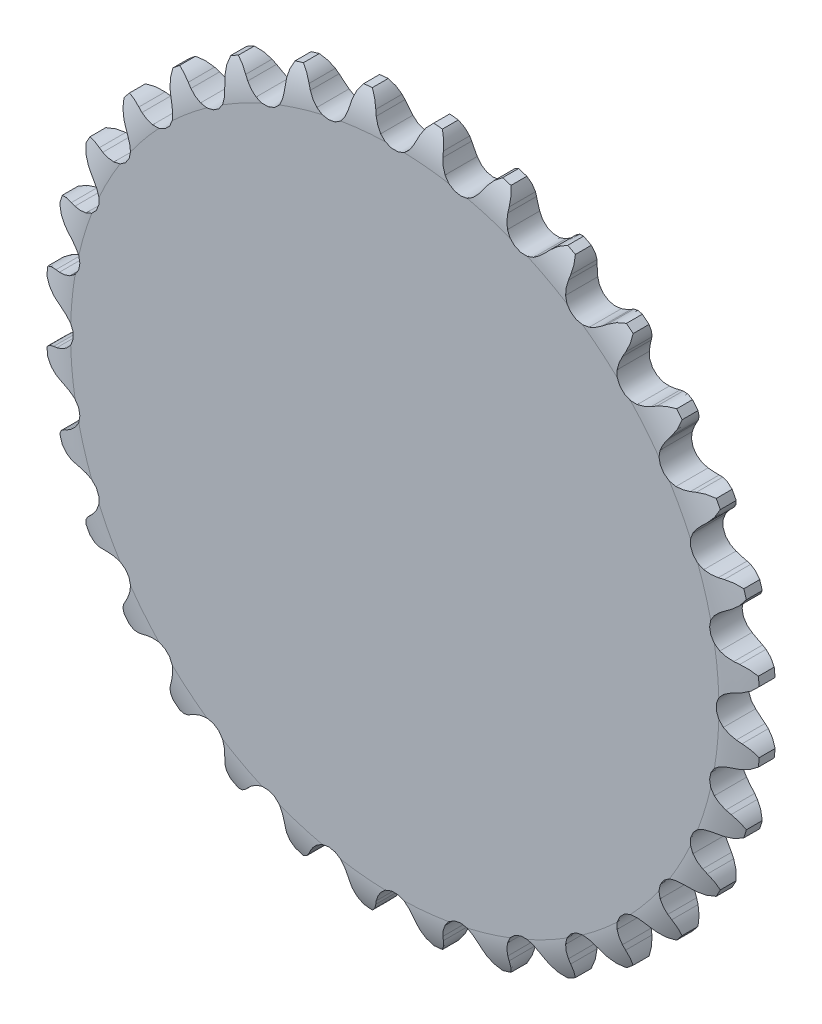
# Autodesk Inventor part: Roller Chain Sprocket1
Saved by Autodesk Inventor 2016 SP1 (Build 200210100, 210)
## iProperties
Created: 2016-02-12
Part Number: Roller Chain Sprocket1
Material: Steel
Document SubType Name: Modeling
Designer: steele
Density: 1 g/cm^3
Appearance: Steel
CustomPartVersion: 1
Author: steele
Autodesk Inventor part; units mm, degrees
ref_plane "YZ Plane" through (0, 0, 0) normal (1, 0, 0) x (0, 1, 0)
ref_plane "XZ Plane" through (0, 0, 0) normal (0, 1, 0) x (-1, 0, 0)
ref_plane "XY Plane" through (0, 0, 0) normal (0, 0, 1) x (1, 0, 0)
sketch "Theoretical Tooth Profile" plane through (0, 0, 0) normal (0, 0, 1) x (1, 0, 0)
  circle A0 centre (0, 0) radius 32.3923 construction
  line L0 (0, 0) -> (0, 32.3923) construction
  line L1 (0, 0) -> (6.3194, 31.7699) construction
  circle A1 centre (0, 0) radius 34.1413
  arc A2 (-1.3578, 31.3738) -> (1.3578, 31.3738) centre (0, 32.3923) ccw
  line L2 (0, 32.3923) -> (6.3194, 31.7699) construction
  line L3 (0, 32.3923) -> (2.1131, 33.9774) construction
  line L4 (2.1131, 33.9774) -> (-1.9477, 32.449) construction
  arc A3 (2.9335, 34.0151) -> (2.1088, 32.877) centre (4.6005, 31.9392) ccw
  arc A4 (-2.1088, 32.877) -> (-2.9335, 34.0151) centre (-4.6005, 31.9392) ccw
  line L5 (-4.6005, 31.9392) -> (-2.1088, 32.877) construction
  arc A5 (-1.9477, 32.449) -> (-1.3578, 31.3738) centre (2.1131, 33.9774) ccw
  line L6 (-1.9477, 32.449) -> (-2.1088, 32.877)
  arc A6 (1.3578, 31.3738) -> (1.9477, 32.449) centre (-2.1131, 33.9774) ccw
  line L7 (2.1088, 32.877) -> (1.9477, 32.449)
  line L8 (0, 0) -> (3.3464, 33.9769) construction
  point P0 (3.1597, 32.0811)
  dimension "d0" = 64.7846
  dimension "d2" = 11.25
  dimension "d3" = 1.6973
  dimension "d10" = 126.875
  dimension "d11" = 16.25
  dimension "d12" = 2.6416
  dimension "d13" = 4.339
  dimension "d14" = 4.6228
  dimension "d23" = 1.905
  constraints: 18 end point, 15 point on circle, 7 centre point, 3 coincident, 3 point on line, 3 symmetric about line, 3 tangent, 1 equal radius, 1 midpoint, 1 parallel, 1 vertical, 1 other
  measures "d0" diameter of A0
  measures "d2" angle of L1 L0
  measures "d3" radius of A2
  measures "d10" angle of L3 L0
  measures "d11" angle of L4 L3
  measures "d12" distance of L2.start L3.end
  measures "d13" distance of L3.end L4.end
  measures "d14" distance of A3.centre L0.end
  measures "d23" distance from line of L8.end L2
sketch "Tooth Profile" plane through (0, 0, 0) normal (0, 0, 1) x (1, 0, 0)
  circle A0 centre (0, 0) radius 34.1413 projected
  line L0 (0, 0) -> (0, 32.3923) construction
  line L1 (0, 32.3923) -> (1.5803, 31.7728) construction
  arc A1 (-1.5803, 31.7728) -> (1.5803, 31.7728) centre (0, 32.3923) ccw
  line L2 (-1.5803, 31.7728) -> (0, 32.3923) construction
  arc A2 (-1.5803, 31.7728) -> (-2.7217, 34.0327) centre (-14.1231, 26.8557) ccw
  arc A3 (2.7217, 34.0327) -> (1.5803, 31.7728) centre (14.1231, 26.8557) ccw
  dimension "d44" = 137.188
  dimension "d45" = 1.6973
  dimension "d46" = 13.4722
  constraints: 8 point on circle, 7 end point, 3 centre point, 2 tangent, 1 coincident, 1 equal radius, 1 symmetric about line, 1 vertical
  measures "d44" angle of L1 L2
  measures "d45" radius of A1
  measures "d46" radius of A3
sketch "Section Profile" plane through (0, 0, 0) normal (1, 0, 0) x (0, 1, 0)
  line L0 (34.1413, 0) -> (-34.1413, 0) projected
  line L1 (28.4263, 1.5526) -> (-28.4263, 1.5526)
  line L2 (-28.4263, 1.5526) -> (-28.4263, -1.5526)
  line L3 (-28.4263, -1.5526) -> (28.4263, -1.5526)
  line L4 (28.4263, -1.5526) -> (28.4263, 1.5526)
  line L5 (28.4263, 1.5526) -> (34.1413, 1.5526) construction
  line L6 (34.1413, 1.5526) -> (34.1413, -1.5526) construction
  line L7 (34.1413, -1.5526) -> (28.4263, -1.5526) construction
  line L8 (28.4263, -1.5526) -> (28.4263, 1.5526)
  arc A0 (34.1413, 0.7588) -> (30.9655, 1.5526) centre (30.9655, -5.1975) ccw
  arc A1 (30.9655, -1.5526) -> (34.1413, -0.7588) centre (30.9655, 5.1975) ccw
  line L9 (30.9655, 1.5526) -> (0, 1.5526)
  line L10 (0, 1.5526) -> (0, -1.5526)
  line L11 (0, -1.5526) -> (30.9655, -1.5526)
  line L12 (0, 1.5526) -> (0, -1.5526)
  line L13 (34.1413, 0.7588) -> (34.1413, -0.7588)
  point P0 (0, 0)
  point P1 (0, 0)
  dimension "d30" = 3.1052
  dimension "d31" = 56.8526
  dimension "d32" = 3.1052
  dimension "d33" = 0.7937
  dimension "d34" = 6.75
  dimension "d43" = 1.5526
  constraints: 26 end point, 7 midpoint, 5 perpendicular, 4 parallel, 4 point on circle, 3 point on line, 3 symmetric about line, 2 centre point, 2 horizontal, 2 tangent, 1 collinear, 1 other
  measures "d30" distance between parallel lines of L7 L5
  measures "d31" distance between parallel lines of L2 L4
  measures "d32" distance between parallel lines of L3 L1
  measures "d33" distance from line of L13.start L5
  measures "d34" radius of A0
  measures "d43" distance between parallel lines of L3 L0
revolve "Shroud" add sketch "Section Profile" angle 360 about axis through (0, 0, 1.5526) along (0, 0, -1) contours L10 L3 L2 L0 | L0 L2 L1 L10
revolve "Strand" add sketch "Section Profile" angle 360 about axis through (0, 0, 1.5526) along (0, 0, -1) contours L13 A1 L11 L4 L0 | L0 L4 L9 A0 L13 | L4 L3 L10 L0 | L0 L10 L1 L4
pattern_of_one "Strand Pattern"
extrude "Theoretical Tooth" cut sketch "Theoretical Tooth Profile" along normal through all both and the other way through all contours A3 L7 A6 A2 A5 L6 A4 A1 picked at (-0.3263, 32.5178)
extrude "Tooth" [suppressed]
pattern_circular "Tooth Pattern" count 32 over 360 about axis through (0, 0, -10) along (0, 0, 1) of "Theoretical Tooth"
ref_plane "Timing Plane" through (0, 32.3923, 0) normal (1, 0, 0) x (0, 1, 0)
equation "\"d3\" = 0.5 * da_Dr + da_SC"
equation "\"d12\" = 0.8 * da_Dr"
equation "\"d13\" = 1.3 * da_Dr + da_SC"
equation "\"d14\" = 1.4 * da_Dr"
equation "\"d23\" = da_Ha"
equation "\"d44\" = da_Alfa"
equation "\"d45\" = da_Ri"
equation "\"d46\" = da_Re"
equation "\"d30\" = da_Bf"
equation "\"d31\" = da_Ds"
equation "\"d32\" = da_Bs"
equation "\"d33\" = da_Ba"
equation "\"d34\" = da_Rx"
equation "\"d40\" = da_pt"
equation "\"form_type\" = 0"
equation "\"da_p\" = 6.35"
equation "\"da_Dr\" = 3.302"
equation "\"da_SC\" = 0.04636"
equation "\"da_Ha\" = 1.905"
equation "\"da_pt\" = 6.4008"
equation "\"da_Bf\" = 3.10515"
equation "\"da_Ba\" = 0.79375"
equation "\"da_Rx\" = 6.75005"
equation "\"da_Ra\" = 0.254"
equation "\"da_Bs\" = 3.10515"
equation "\"da_Ds\" = 56.85263"
equation "\"da_Re\" = 13.47216"
equation "\"da_Ri\" = 1.69735"
equation "\"da_Alfa\" = 137.188deg"
body "Solid1"
